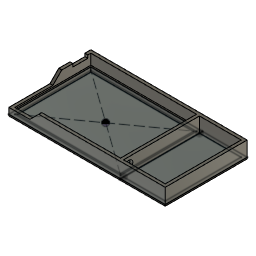
7SegMultiDemoCase v1 (Autodesk Fusion 360 design; units mm, degrees)
Autodesk Fusion 360 part; units mm, degrees
sketch "Sketch1" plane through (0, 0, 0) normal (0, 0, 1) x (1, 0, 0)
  line L0 (35.5, -25.5) -> (-35.5, -25.5)
  line L1 (-35.5, -25.5) -> (-35.5, 25.5)
  line L2 (-35.5, 25.5) -> (35.5, 25.5)
  line L3 (35.5, 25.5) -> (35.5, -25.5)
  line L4 (35.5, -25.5) -> (-35.5, 25.5) construction
  line L5 (-35.5, -25.5) -> (35.5, 25.5) construction
  line L6 (34.5, -24.5) -> (-34.5, -24.5)
  line L7 (-34.5, -24.5) -> (-34.5, 24.5)
  line L8 (-34.5, 24.5) -> (34.5, 24.5)
  line L9 (34.5, 24.5) -> (34.5, -24.5)
  line L10 (-37.5, -27.5) -> (-37.5, 27.5)
  line L11 (-37.5, 27.5) -> (37.5, 27.5)
  line L12 (37.5, 27.5) -> (37.5, -27.5)
  line L13 (37.5, -27.5) -> (-37.5, -27.5)
  line L14 (37.5, -27.5) -> (67.5, -27.5)
  line L15 (67.5, -27.5) -> (67.5, 27.5)
  line L16 (67.5, 27.5) -> (37.5, 27.5)
  line L17 (37.5, 27.5) -> (37.5, -27.5)
  line L18 (37.5, -25.5) -> (65.5, -25.5)
  line L19 (65.5, -25.5) -> (65.5, 25.5)
  line L20 (65.5, 25.5) -> (37.5, 25.5)
  dimension "d1" = 71
  dimension "d2" = 51
  dimension "d3" = 1
  dimension "d4" = -2
  dimension "d5" = 30
  dimension "d6" = 55
  dimension "d7" = -2
  constraint horizontal L0
  constraint perpendicular L0 L1
  constraint parallel L0 L2
  constraint parallel L1 L3
  constraint coincident L4 origin
  constraint coincident L5 origin
  constraint horizontal L14
  constraint vertical L15
  constraint horizontal L16
  constraint vertical L17
  measures "d1" distance of L1.end L2.end
  measures "d2" distance of L0.end L1.end
  measures "d5" distance of L12.end L14.end
  measures "d6" distance of L12.end L11.end
extrude "Extrude1" add sketch "Sketch1" along normal blind 10 contours L10 L11 L12 L13 L17 | L12 L14 L15 L16 L17 L18 L19 L20
extrude "Extrude2" add sketch "Sketch1" against normal blind 1 contours L0 L1 L2 L3 | L6 L7 L8 L9 | L10 L11 L12 L13 L17 | L12 L14 L15 L16 L17 L18 L19 L20 | L12 L17 L18 L19 L20
extrude "Extrude3" add sketch "Sketch1" along normal blind 3 contours L0 L1 L2 L3
hole "Hole1" at (37.5, -21.7224, 5.415) direction (-1, 0, 0) diameter 5 depth 5 tip angle 118
sketch "Sketch2" plane through (0, 0, 10) normal (0, 0, 1) x (-1, 0, 0)
  line L0 (35.5, -25.5) -> (-35.5, -25.5)
  line L1 (-35.5, -25.5) -> (-35.5, 25.5)
  line L2 (-35.5, 25.5) -> (35.5, 25.5)
  line L3 (35.5, 25.5) -> (35.5, -25.5)
  line L4 (-37.5, -25.5) -> (-65.5, -25.5)
  line L5 (-65.5, -25.5) -> (-65.5, 25.5)
  line L6 (-65.5, 25.5) -> (-37.5, 25.5)
  line L7 (-37.5, 25.5) -> (-37.5, -25.5)
  line L8 (37.5, 27.5) -> (-67.5, 27.5)
  line L9 (-67.5, 27.5) -> (-67.5, -27.5)
  line L10 (-67.5, -27.5) -> (37.5, -27.5)
  line L11 (37.5, -27.5) -> (37.5, 27.5)
  line L12 (37.5, 0) -> (23.5, 0)
  line L13 (23.5, 0) -> (23.5, 27.5)
  line L14 (23.5, 27.5) -> (37.5, 27.5)
  line L15 (37.5, 27.5) -> (37.5, 0)
  dimension "d17" = 14
  constraint horizontal L12
  constraint vertical L13
  constraint horizontal L14
  constraint vertical L15
  constraint midpoint L11 L12.start
  measures "d17" distance of L12.start L12.end
extrude "Extrude4" cut sketch "Sketch2" against normal blind 6 contours L2 L3 L8 L11 L12 L13 L14 L15
sketch "Sketch3" plane through (0, -27.5, 0) normal (0, -1, 0) x (1, 0, 0)
  line L0 (-23.5, 4) -> (-37.5, 4)
  line L1 (-37.5, 4) -> (-37.5, -1)
  line L2 (-37.5, -1) -> (67.5, -1)
  line L3 (67.5, -1) -> (67.5, 10)
  line L4 (67.5, 10) -> (-23.5, 10)
  line L5 (-23.5, 10) -> (-23.5, 4)
  line L6 (-23.5, 4) -> (0.8403, 28.3403)
  line L7 (-23.5, 4) -> (10.9224, 4) construction
  line L8 (-17.5, 10) -> (-17.5, 4)
  line L9 (-23.5, 4) -> (-17.5, 4)
  dimension "d23" = 45
  constraint horizontal L7
  constraint coincident L0.start L5.end
  constraint coincident L6 L8.start
  constraint coincident L4 L8.start
  constraint coincident L7 L8.end
  constraint perpendicular L7 L8
  measures "d23" angle of L6 L7
extrude "Extrude5" cut sketch "Sketch3" against normal blind 8 contours L4 L5 L6
sketch "Sketch4" plane through (-37.5, 0, 0) normal (-1, 0, 0) x (0, -1, 0)
  line L0 (27.5, 4) -> (0, 4)
  line L1 (0, 4) -> (0, 10)
  line L2 (0, 10) -> (-27.5, 10)
  line L3 (-27.5, 10) -> (-27.5, -1)
  line L4 (-27.5, -1) -> (27.5, -1)
  line L5 (27.5, -1) -> (27.5, 4)
  line L6 (-27.5, 10) -> (-23.5, 10)
  line L7 (-23.5, 10) -> (-13.5, 10)
  line L8 (0, 4) -> (-6, 10)
  line L9 (0, 4) -> (8.4853, 4) construction
  line L10 (0, 4) -> (-27.5, 4)
  line L11 (-6, 10) -> (-6, 4)
  line L12 (-13.5, 10) -> (-13.5, 8)
  line L13 (-23.5, 10) -> (-23.5, 8)
  line L14 (-23.5, 8) -> (-13.5, 8)
  dimension "d26" = 4
  dimension "d27" = 10
  dimension "d28" = 135
  dimension "d29" = 2
  constraint coincident L2.end L3.start
  constraint perpendicular L3 L6
  constraint perpendicular L3 L7
  constraint horizontal L9
  constraint coincident L0.end L1.start
  constraint coincident L2 L8.end
  constraint coincident L3 L10.end
  constraint perpendicular L3 L10
  constraint coincident L10 L11.end
  constraint perpendicular L10 L11
  constraint perpendicular L2 L12
  constraint perpendicular L6 L13
  measures "d26" distance of L2.end L6.end
  measures "d27" distance of L6.end L7.end
  measures "d28" angle of L8 L9
  measures "d29" distance of L6.end L13.end
extrude "Extrude6" cut sketch "Sketch4" against normal blind 5.5 contours L1 L2 L8 | L2 L7 L12 L13 L14
named bodies: "7SegMultiDemo"
